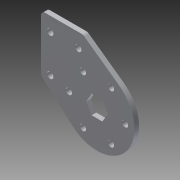
# Autodesk Inventor part: Hex Shaft Connector Pivot
Saved by Autodesk Inventor 2014 (Build 180170000, 170)
## iProperties
Created: 2014-02-11
Part Number: Hex Shaft Connector Pivot
Material: Aluminum 6061
Document SubType Name: Modeling
Designer: Michael
Density: 2.71 g/cm^3
Appearance: Aluminum - Flat
Author: Michael
Autodesk Inventor part; units mm, degrees
ref_plane "YZ Plane" through (0, 0, 0) normal (1, 0, 0) x (0, 1, 0)
ref_plane "XZ Plane" through (0, 0, 0) normal (0, 1, 0) x (-1, 0, 0)
ref_plane "XY Plane" through (0, 0, 0) normal (0, 0, 1) x (1, 0, 0)
sketch "Sketch1" plane through (0, 0, 0) normal (0, 0, 1) x (1, 0, 0)
  arc A0 (-16.9333, -18.932) -> (14.8097, 20.6357) centre (0, 0) ccw
  circle A1 centre (9.525, 16.4978) radius 2.0828
  circle A2 centre (-9.525, 16.4978) radius 2.0828
  circle A3 centre (-19.05, 0) radius 2.0828
  circle A4 centre (-9.525, -16.4978) radius 2.0828
  circle A5 centre (9.525, -16.4978) radius 2.0828
  circle A6 centre (19.05, 0) radius 2.0828
  line L0 (0, 0) -> (-66.675, 0) construction
  line L1 (-16.9333, -18.932) -> (-38.1, 0)
  line L2 (-38.1, 0) -> (-38.1, 38.1)
  line L3 (-38.1, 38.1) -> (-9.525, 38.1)
  circle A7 centre (-31.75, 28.575) radius 2.159
  circle A8 centre (-31.75, 3.175) radius 2.159
  line L4 (14.8097, 20.6357) -> (-9.525, 38.1)
  circle A9 centre (-12.7, 28.575) radius 2.159
  line L5 (3.6662, 6.35) -> (7.3323, 0)
  line L6 (7.3323, 0) -> (3.6662, -6.35)
  line L7 (3.6662, -6.35) -> (-3.6662, -6.35)
  line L8 (-3.6662, -6.35) -> (-7.3323, 0)
  line L9 (-7.3323, 0) -> (-3.6662, 6.35)
  line L10 (-3.6662, 6.35) -> (3.6662, 6.35)
  dimension "d0" = 50.8
  dimension "d2" = 4.1656
  dimension "d3" = 19.05
  dimension "d6" = 360
  dimension "d13" = 38.1
  dimension "d14" = 38.1
  dimension "d15" = 9.525
  dimension "d16" = 6.35
  dimension "d19" = 25.4
  dimension "d31" = 4.318
  dimension "d32" = 28.575
  dimension "d35" = 19.05
  dimension "d41" = 12.7
  constraints: 22 end point, 10 centre point, 3 coincident, 3 horizontal, 3 point on line, 2 perpendicular, 2 point on circle, 2 tangent, 1 vertical, 30 other
  measures "d0" diameter of A0
  measures "d2" diameter of A1
  measures "d3" distance of A1.centre point (0, 0)
  measures "d13" distance of L1.end point (0, 0)
  measures "d14" distance of L1.end L2.end
  measures "d15" distance from line of L3 A7.centre
  measures "d16" distance from line of L2 A7.centre
  measures "d19" distance of A7.centre A8.centre
  measures "d31" diameter of A7
  measures "d32" distance from line of L3.end L2
  measures "d35" distance of A7.centre A9.centre
  measures "d41" distance between parallel lines of L7 L10
extrude "Extrusion1" add sketch "Sketch1" along normal blind 3.175
fillet "Fillet1" radius 3.175 3 edges at (-38.1, 0, 1.5875) (-38.1, 38.1, 1.5875) (-9.525, 38.1, 1.5875)
body "Solid1"
